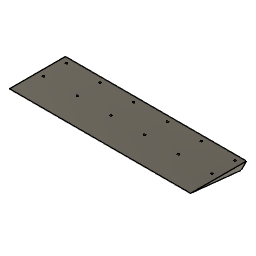
Case Stand v7 (Autodesk Fusion 360 design; units mm, degrees)
Autodesk Fusion 360 part; units mm, degrees
sketch "Sketch1" plane through (0, 0, 0) normal (0, 0, 1) x (1, 0, 0)
  line L0 (-217, 72) -> (217, 72)
  line L1 (217, 72) -> (217, -62)
  line L2 (217, -62) -> (-217, -62)
  line L3 (-217, -62) -> (-217, 72)
  constraint horizontal L0
  constraint vertical L1
  constraint horizontal L2
  constraint vertical L3
extrude "Extrude4" add sketch "Sketch1" against normal blind 230
sketch "Sketch4" plane through (-217, 0, 0) normal (-1, 0, 0) x (0, -1, 0)
  line L0 (62, 0) -> (-72, 0)
  line L1 (-72, 0) -> (-72, -230)
  line L2 (-72, -230) -> (62, -230)
  line L3 (62, -230) -> (62, 0)
  line L4 (62, 0) -> (-29, 0) construction
  line L5 (-72, 0) -> (-59.2555, -12.7445)
  line L6 (-72, 0) -> (-53.9766, 0) construction
  line L7 (62, 0) -> (-59.2555, -12.7445)
  line L8 (62, 0) -> (-59.9234, 0) construction
  dimension "d30" = 45
  dimension "d31" = 6
  constraint horizontal L4
  constraint coincident L0.start L3.end
  constraint horizontal L6
  constraint coincident L0.end L1.start
  constraint horizontal L8
  constraint coincident L5 L7.end
  measures "d30" angle of L5 L6
  measures "d31" angle of L7 L8
extrude "Extrude5" cut sketch "Sketch4" against normal blind 520 contours L1 L2 L3 L5 L7
sketch "Sketch5" plane through (0, 0, 0) normal (0, 0, 1) x (-1, 0, 0)
  line L0 (217, 62) -> (-217, 62)
  line L1 (-217, 62) -> (-217, -72)
  line L2 (-217, -72) -> (217, -72)
  line L3 (217, -72) -> (217, 62)
  circle A0 centre (202, -59.25) radius 2.25
  circle A1 centre (121.2, -59.25) radius 2.25
  circle A2 centre (40.4, -59.25) radius 2.25
  circle A3 centre (-40.4, -59.25) radius 2.25
  circle A4 centre (-121.2, -59.25) radius 2.25
  circle A5 centre (-202, -59.25) radius 2.25
  circle A6 centre (202, -4.5) radius 2.25
  circle A7 centre (121.2, -4.5) radius 2.25
  circle A8 centre (40.4, -4.5) radius 2.25
  circle A9 centre (-40.4, -4.5) radius 2.25
  circle A10 centre (-121.2, -4.5) radius 2.25
  circle A11 centre (-202, -4.5) radius 2.25
  dimension "d34" = 4.5
  dimension "d35" = 12.75
  dimension "d36" = 15
  dimension "d39" = -404
  dimension "d40" = 0
  dimension "d41" = 4.5
  dimension "d42" = 66.5
  dimension "d43" = 15
  dimension "d46" = -404
  dimension "d47" = 0
  measures "d34" diameter of A0
  measures "d35" distance of L2 A0.centre
  measures "d36" distance of L3 A0.centre
  measures "d41" diameter of A6
  measures "d42" distance of L0 A6.centre
  measures "d43" distance of L3 A6.centre
extrude "Extrude6" cut sketch "Sketch5" against normal blind 6 contours A0 | A1 | A2 | A3 | A4 | A5 | A6 | A7 | A8 | A9 | A10 | A11
